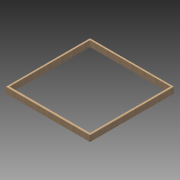
# Autodesk Inventor part: Wände
Saved by Autodesk Inventor 2013 SP1 (Build 170176100, 176)
## iProperties
Created: 2012-12-07
Part Number: Wände
Material: Esche
Document SubType Name: Modeling
Designer: Sebastian
Density: 1 g/cm^3
Author: Sebastian
Autodesk Inventor part; units mm, degrees
ref_plane "YZ Plane" through (0, 0, 0) normal (1, 0, 0) x (0, 1, 0)
ref_plane "XZ Plane" through (0, 0, 0) normal (0, 1, 0) x (-1, 0, 0)
ref_plane "XY Plane" through (0, 0, 0) normal (0, 0, 1) x (1, 0, 0)
sketch "Skizze Helper" plane through (0, 0, 0) normal (0, 0, 1) x (1, 0, 0)
  line L0 (-210, -210) -> (210, -210) construction
  line L1 (210, -210) -> (210, 210) construction
  line L2 (210, 210) -> (-210, 210) construction
  line L3 (-210, 210) -> (-210, -210) construction
  line L4 (-210, -210) -> (210, 210) construction
  line L5 (210, -210) -> (-210, 210) construction
  line L6 (201, -201) -> (-201, -201) construction
  line L7 (-201, -201) -> (-201, 201) construction
  line L8 (-201, 201) -> (201, 201) construction
  line L9 (201, 201) -> (201, -201) construction
  line L10 (201, -201) -> (-201, 201) construction
  line L11 (-201, -201) -> (201, 201) construction
  point P0 (0, 0)
  dimension "d0" = 420
  dimension "d1" = 420
  dimension "d2" = 402
  dimension "d3" = 402
  constraints: 24 end point, 4 midpoint, 4 parallel, 2 horizontal, 2 perpendicular
  measures "d0" distance of L2.end L1.end
  measures "d1" distance of L1.end L0.end
  measures "d2" distance of L7.end L8.end
  measures "d3" distance of L6.end L7.end
sketch "Skizze8" plane through (0, 0, 0) normal (0, 0, 1) x (1, 0, 0)
  line L0 (-210, -210) -> (210, -210)
  line L1 (210, -210) -> (210, -201)
  line L2 (210, -201) -> (-210, -201)
  line L3 (-210, -201) -> (-210, -210)
  point P0 (0, 0)
  constraints: 8 end point, 2 parallel, 1 horizontal, 1 perpendicular
extrude "Extrusion7" add sketch "Skizze8" against normal blind 40
sketch "Skizze9" plane through (0, 0, 0) normal (0, 0, 1) x (1, 0, 0)
  line L0 (-201, -201) -> (-210, -201)
  line L1 (-210, -201) -> (-210, 201)
  line L2 (-210, 201) -> (-201, 201)
  line L3 (-201, 201) -> (-201, -201)
  point P0 (0, 0)
  constraints: 8 end point, 2 parallel, 1 horizontal, 1 perpendicular
extrude "Extrusion8" add sketch "Skizze9" against normal blind 40 separate body
mirror "Spiegeln5" about plane through (0, 0, 0) normal (0, 1, 0) of "Extrusion7" bodies 1
mirror "Spiegeln6" about plane through (0, 0, 0) normal (1, 0, 0) of "Extrusion8" bodies 2
chamfer "Fase2" distance 1 angle 45 4 edges at (210, -210, -20) (-210, -210, -20) (-210, 210, -20) (210, 210, -20)
chamfer "Fase3" distance 1 angle 45 8 edges at (0, -210, 0) (0, 210, 0) (210, 205, 0) (-210, 205, 0) (210, -205, 0) (-210, -205, 0) (-210, 0, 0) (210, 0, 0)
chamfer "Fase4" distance 1 angle 45 1 edges at (210, 201, -20.5)
chamfer "Fase5" distance 1 angle 45 1 edges at (210, -201, -20.5)
chamfer "Fase6" distance 1 angle 45 1 edges at (-210, -201, -20.5)
chamfer "Fase7" distance 1 angle 45 1 edges at (-210, 201, -20.5)
